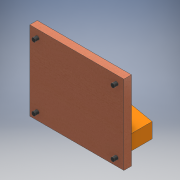
# Autodesk Inventor part: basic plate
Saved by Autodesk Inventor 2018 (Build 220112000, 112)
## iProperties
Created: 2017-10-09
Part Number: basic plate
Material: Generic
Document SubType Name: Modeling
Designer: HP
Density: 1 g/cm^3
Appearance: Default
Author: HP
Autodesk Inventor part; units mm, degrees
ref_plane "YZ Plane" through (0, 0, 0) normal (1, 0, 0) x (0, 1, 0)
ref_plane "XZ Plane" through (0, 0, 0) normal (0, 1, 0) x (-1, 0, 0)
ref_plane "XY Plane" through (0, 0, 0) normal (0, 0, 1) x (1, 0, 0)
sketch "Sketch1" plane through (0, 0, 0) normal (0, 1, 0) x (-1, 0, 0)
  line L0 (0, -210) -> (-250, -210)
  line L1 (-250, -210) -> (-250, 0)
  line L2 (-250, 0) -> (0, 0)
  line L3 (0, 0) -> (0, -210)
  dimension "d0" = 250
  dimension "d1" = 210
  constraints: 8 end point, 2 parallel, 1 coincident, 1 horizontal, 1 perpendicular
  measures "d0" distance of L1.end L2.end
  measures "d1" distance of L0.end L1.end
extrude "Extrusion1" add sketch "Sketch1" along normal blind 20
sketch "Sketch2" plane through (0, 0, 0) normal (0, -1, 0) x (1, 0, 0)
  circle A0 centre (20, -20) radius 5
  line L0 (0, -210) -> (250, -210) construction
  line L1 (250, -210) -> (250, 0) construction
  line L2 (250, 0) -> (0, 0) construction
  line L3 (0, 0) -> (0, -210) construction
  circle A1 centre (20, -190) radius 5
  circle A2 centre (230, -20) radius 5
  circle A3 centre (230, -190) radius 5
  dimension "d4" = 10
  dimension "d5" = 20
  dimension "d6" = 20
  dimension "d7" = 10
  dimension "d8" = 20
  dimension "d9" = 20
  dimension "d10" = 10
  dimension "d11" = 10
  dimension "d12" = 20
  dimension "d13" = 20
  dimension "d14" = 20
  dimension "d15" = 20
  constraints: 4 centre point
  measures "d4" diameter of A0
  measures "d5" horizontal distance of A0.centre point (0, 0)
  measures "d6" horizontal distance of A0.centre point (0, 0)
  measures "d7" diameter of A1
  measures "d8" distance from line of L0 A1.centre
  measures "d9" horizontal distance of L0.start A1.centre
  measures "d10" diameter of A2
  measures "d11" diameter of A3
  measures "d12" distance from line of A3.centre L1
  measures "d13" horizontal distance of L0.end A3.centre
  measures "d14" horizontal distance of L1.end A2.centre
  measures "d15" horizontal distance of L1.end A2.centre
extrude "Extrusion2" add sketch "Sketch2" along normal blind 10
sketch "Sketch3" plane through (0, 20, 0) normal (0, 1, 0) x (1, 0, 0)
  line L0 (245, 180) -> (245, 140)
  line L1 (245, 140) -> (153.1686, 120.843)
  line L2 (245, 180) -> (153.1686, 199.157)
  arc A0 (153.1686, 199.157) -> (153.1686, 120.843) centre (145, 160) ccw
  line L3 (250, 210) -> (0, 210) construction
  line L4 (0, 210) -> (0, 0) construction
  line L5 (0, 0) -> (250, 0) construction
  line L6 (250, 0) -> (250, 210) construction
  line L7 (250, 0) -> (250, 210) construction
  line L8 (245, 160) -> (145, 160) construction
  dimension "d21" = 5
  dimension "d22" = 30
  dimension "d23" = 40
  dimension "d24" = 80
  dimension "d25" = 100
  constraints: 8 end point, 2 point on circle, 1 centre point, 1 coincident, 1 horizontal, 1 midpoint, 1 parallel, 1 tangent, 1 vertical, 1 other
  measures "d21" distance between parallel lines of L6 L0
  measures "d22" distance from line of L0.start L3
  measures "d23" distance of L0.end L0.start
  measures "d24" diameter of A0
  measures "d25" distance from line of A0.centre L0
extrude "Extrusion3" add sketch "Sketch3" along normal blind 60
equation "\"d6\" = d5"
equation "\"d8\" = d5"
equation "\"d9\" = d5"
equation "\"d12\" = d5"
equation "\"d13\" = d5"
equation "\"d14\" = d5"
equation "\"d15\" = d5"
body "Solid1"
